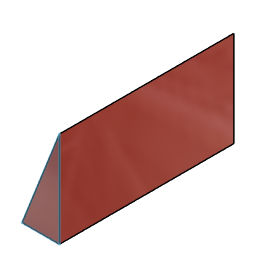
Triangular Prism v5 (Autodesk Fusion 360 design; units mm, degrees)
Autodesk Fusion 360 part; units mm, degrees
sketch "Sketch1" plane through (0, 0, 0) normal (0, 1, 0) x (1, 0, 0)
  line L0 (-27.94, 0) -> (-5.08, 0)
  line L1 (-5.08, 0) -> (-5.08, -58.42)
  line L2 (-5.08, -58.42) -> (-27.94, 0)
  constraint horizontal L0
  constraint perpendicular L0 L1
extrude "Extrude2" add sketch "Sketch1" along normal blind 106.68
